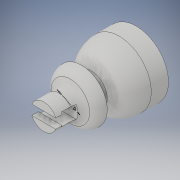
# Autodesk Inventor part: Elektrodenhalter_final_medium_uShapeRound_forCables
Saved by Autodesk Inventor 2018 (Build 220112000, 112)
## iProperties
Part Number: Elektrodenhalter_final_medium_uShapeRound_forCables
Material: Generisch
Document SubType Name: Modeling
Designer: Timo
Density: 1 g/cm^3
Appearance: Vorgabe
Author: Timo
Autodesk Inventor part; units mm, degrees
ref_plane "YZ Plane" through (0, 0, 0) normal (1, 0, 0) x (0, 1, 0)
ref_plane "XZ Plane" through (0, 0, 0) normal (0, 1, 0) x (-1, 0, 0)
ref_plane "XY Plane" through (0, 0, 0) normal (0, 0, 1) x (1, 0, 0)
sketch "Skizze1" plane through (0, 0, 0) normal (0, 1, 0) x (-1, 0, 0)
  circle A0 centre (0, 0) radius 4
  dimension "d0" = 8
  constraints: 1 centre point, 1 coincident
  measures "d0" diameter of A0
extrude "Extrusion1" add sketch "Skizze1" along normal blind 2
fillet "Rundung1" radius 2 1 edges at (4, 0, 0)
sketch "Skizze2" plane through (0, 2, 0) normal (0, 1, 0) x (1, 0, 0)
  circle A0 centre (0, 0) radius 2.5
  dimension "d4" = 5
  constraints: 1 centre point, 1 coincident
  measures "d4" diameter of A0
extrude "Extrusion2" add sketch "Skizze2" along normal blind 1.5
sketch "Skizze3" plane through (0, 3.5, 0) normal (0, 1, 0) x (1, 0, 0)
  circle A0 centre (0, 0) radius 5
  dimension "d7" = 10
  constraints: 1 centre point, 1 coincident
  measures "d7" diameter of A0
extrude "Extrusion3" add sketch "Skizze3" along normal blind 5
sketch "Skizze5" plane through (0, 8.5, 0) normal (0, 1, 0) x (1, 0, 0)
  circle A0 centre (0, 0) radius 5
  dimension "d13" = 10
  constraints: 1 centre point, 1 coincident
  measures "d13" diameter of A0
extrude "Extrusion5" add sketch "Skizze5" along normal blind 2
sketch "Skizze6" plane through (0, 10.5, 0) normal (0, 1, 0) x (1, 0, 0)
  circle A0 centre (0, 0) radius 4.25
  dimension "d16" = 8.5
  constraints: 1 centre point, 1 coincident
  measures "d16" diameter of A0
extrude "Extrusion6" cut sketch "Skizze6" against normal blind 2
sketch "Skizze8" plane through (0, 8.5, 0) normal (0, 1, 0) x (1, 0, 0)
  circle A0 centre (0, 0) radius 0.8
  dimension "d19" = 1.6
  constraints: 1 centre point, 1 coincident
  measures "d19" diameter of A0
extrude "Extrusion7" add sketch "Skizze8" along normal blind 1.1
fillet "Rundung2" radius 5 1 edges at (-5, 3.5, 0)
sketch "Skizze11" plane through (0, 0, 0) normal (0, -1, 0) x (1, 0, 0)
  circle A0 centre (0, 0) radius 2
  dimension "d23" = 4
  constraints: 1 centre point, 1 coincident
  measures "d23" diameter of A0
sketch "Skizze12" plane through (0, 0, 0) normal (0, -1, 0) x (1, 0, 0)
  circle A0 centre (0, 0) radius 2
  dimension "d24" = 4
  constraints: 1 centre point, 1 coincident
  measures "d24" diameter of A0
extrude "Extrusion8" add sketch "Skizze12" along normal blind 2.85
sketch "Skizze13" plane through (0, -2.85, 0) normal (0, -1, 0) x (1, 0, 0)
  line L0 (-2.5639, -1.0002) -> (2.5639, -1.0002)
  line L1 (2.5639, -1.0002) -> (2.5639, 1.0002)
  line L2 (2.5639, 1.0002) -> (-2.5639, 1.0002)
  line L3 (-2.5639, 1.0002) -> (-2.5639, -1.0002)
  line L4 (-2.5639, -1.0002) -> (2.5639, 1.0002) construction
  line L5 (2.5639, -1.0002) -> (-2.5639, 1.0002) construction
  point P0 (0, 0)
  constraints: 12 end point, 2 midpoint, 2 parallel, 1 horizontal, 1 perpendicular
extrude "Extrusion9" cut sketch "Skizze13" against normal blind 2.15
sketch "Skizze14" plane through (0, -2.85, 0) normal (0, -1, 0) x (1, 0, 0)
  circle A0 centre (0, 0) radius 2
  dimension "d29" = 4
  constraints: 1 centre point, 1 coincident
  measures "d29" diameter of A0
extrude "Extrusion10" add sketch "Skizze14" along normal blind 1
sketch "Skizze15" plane through (0, -3.85, 0) normal (0, -1, 0) x (1, 0, 0)
  line L0 (-3.1829, -0.7502) -> (3.1829, -0.7502)
  line L1 (3.1829, -0.7502) -> (3.1829, 0.7502)
  line L2 (3.1829, 0.7502) -> (-3.1829, 0.7502)
  line L3 (-3.1829, 0.7502) -> (-3.1829, -0.7502)
  line L4 (-3.1829, -0.7502) -> (3.1829, 0.7502) construction
  line L5 (3.1829, -0.7502) -> (-3.1829, 0.7502) construction
  point P0 (0, 0)
  constraints: 12 end point, 2 midpoint, 2 parallel, 1 horizontal, 1 perpendicular
extrude "Extrusion11" cut sketch "Skizze15" against normal blind 1
fillet "Rundung3" radius 2 2 edges at (0, 0, 2.0001) (0, 0, -2.0001)
